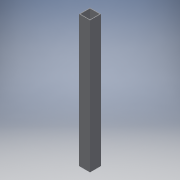
# Autodesk Inventor part: frontrollcage
Saved by Autodesk Inventor 2016 (Build 200138000, 138)
## iProperties
Created: 2016-02-23
Part Number: frontrollcage
Material: Aluminum 6061
Document SubType Name: Modeling
Designer: gus
Density: 2.7 g/cm^3
Appearance: Aluminum - Flat
Author: gus
Autodesk Inventor part; units mm, degrees
ref_plane "YZ Plane" through (0, 0, 0) normal (1, 0, 0) x (0, 1, 0)
ref_plane "XZ Plane" through (0, 0, 0) normal (0, 1, 0) x (-1, 0, 0)
ref_plane "XY Plane" through (0, 0, 0) normal (0, 0, 1) x (1, 0, 0)
sketch "Sketch1" plane through (0, 0, 0) normal (0, 1, 0) x (-1, 0, 0)
  line L0 (0, 0) -> (-25.4, 0)
  line L1 (-25.4, 0) -> (-25.4, -25.4)
  line L2 (-25.4, -25.4) -> (0, -25.4)
  line L3 (0, -25.4) -> (0, 0)
  line L4 (-23.8125, -23.8125) -> (-23.8125, -1.5875)
  line L5 (-23.8125, -1.5875) -> (-1.5875, -1.5875)
  line L6 (-1.5875, -1.5875) -> (-1.5875, -23.8125)
  line L7 (-1.5875, -23.8125) -> (-23.8125, -23.8125)
  dimension "d0" = 25.4
  dimension "d1" = 25.4
  dimension "d2" = 1.5875
  constraints: 16 end point, 4 parallel, 2 perpendicular, 1 horizontal, 3 other
  measures "d0" distance of L2.end L1.end
  measures "d1" distance of L1.end L0.end
  measures "d2" distance between parallel lines of L1 L4
extrude "Extrusion1" add sketch "Sketch1" along normal blind 238.0191
sketch "Sketch2" plane through (25.4, 0, 0) normal (1, 0, 0) x (0, 0, -1)
  line L0 (0, 0) -> (0, 238.0191) projected
  line L1 (0, 0) -> (25.4, 26.3769)
  line L2 (25.4, 0) -> (25.4, 238.0191) projected
  line L3 (0, 0) -> (25.4, 0) projected
  line L4 (25.4, 26.3769) -> (25.4, 0)
  line L5 (25.4, 0) -> (0, 0)
  dimension "d5" = 43.919
  constraints: 6 end point, 1 perpendicular, 1 point on line, 1 vertical
  measures "d5" angle of L0 L1
extrude "Extrusion2" cut sketch "Sketch2" against normal blind 25.4
body "Solid1"
